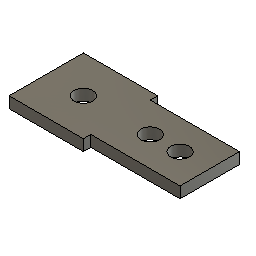
ITEM5-LEGO-ASM v5 (Autodesk Fusion 360 archive; units mm, degrees)
design "ITEM5-LEGO"
Autodesk Fusion 360 part; units mm, degrees
sketch "Sketch1" plane through (0, 0, 0) normal (0, 1, 0) x (1, 0, 0)
  line L0 (10, 10) -> (-10, 10)
  line L1 (-10, 10) -> (-10, -10)
  line L2 (-10, -10) -> (10, -10)
  line L3 (10, -10) -> (10, 10)
  line L4 (10, 10) -> (-10, -10) construction
  line L5 (-10, 10) -> (10, -10) construction
  circle A0 centre (0, 0) radius 2.5
  circle A1 centre (18, 0) radius 2.5
  circle A2 centre (26, 0) radius 2.5
  line L6 (34, 8) -> (10, 8)
  line L7 (10, 8) -> (10, -8)
  line L8 (10, -8) -> (34, -8)
  line L9 (34, -8) -> (34, 8)
  line L10 (34, 8) -> (10, -8) construction
  line L11 (10, 8) -> (34, -8) construction
  point P0 (22, 0)
  dimension "d1" = 20
  dimension "d2" = 20
  dimension "d3" = 5
  dimension "d4" = 5
  dimension "d5" = 5
  dimension "d6" = 8
  dimension "d7" = 8
  dimension "d8" = 24
  dimension "d9" = 16
  dimension "d10" = 12
  constraint perpendicular L0 L1
  constraint parallel L0 L2
  constraint parallel L1 L3
  constraint horizontal L0
  constraint coincident L4 A0.centre
  constraint coincident L5 A0.centre
  constraint coincident A0.centre origin
  constraint perpendicular L6 L7
  constraint parallel L6 L8
  constraint parallel L7 L9
  constraint horizontal L6
  constraint coincident L10 P0
  constraint coincident L11 P0
  measures "d1" distance of L1.end L2.end
  measures "d2" distance of L0.end L1.end
  measures "d3" diameter of A0
  measures "d4" diameter of A1
  measures "d5" diameter of A2
  measures "d6" distance of L3 A1.centre
  measures "d7" distance of A1.centre A2.centre
  measures "d8" distance of L7.end L8.end
  measures "d9" distance of L6.end L7.end
  measures "d10" horizontal distance of L0.start P0
extrude "Extrude1" add sketch "Sketch1" along normal blind 3
